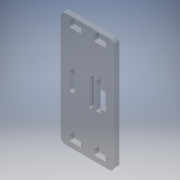
# Autodesk Inventor part: Front_wall
Saved by Autodesk Inventor 2016 (Build 200138000, 138)
## iProperties
Created: 2015-06-25
Part Number: Front_wall
Material: Generic
Document SubType Name: Modeling
Designer: Openlab
Density: 1 g/cm^3
Appearance: Polycarbonate - Clear
Author: Openlab
Autodesk Inventor part; units mm, degrees
ref_plane "YZ Plane" through (0, 0, 0) normal (1, 0, 0) x (0, 1, 0)
ref_plane "XZ Plane" through (0, 0, 0) normal (0, 1, 0) x (-1, 0, 0)
ref_plane "XY Plane" through (0, 0, 0) normal (0, 0, 1) x (1, 0, 0)
sketch "Sketch1" plane through (0, 0, 0) normal (0, 1, 0) x (-1, 0, 0)
  line L0 (15.75, -20.2435) -> (15.75, -42.6397) construction
  line L1 (13.2323, -33.5) -> (6.4845, -33.5) construction
  line L2 (31.5, -64) -> (31.5, -3)
  line L3 (0, -3) -> (0, -64)
  line L4 (28.5, 0) -> (3, 0)
  line L5 (3, -67) -> (28.5, -67)
  line L6 (14.8, -41) -> (13, -41)
  line L7 (13, -41) -> (13, -26)
  line L8 (13, -26) -> (14.8, -26)
  line L9 (14.8, -26) -> (14.8, -41)
  line L10 (26.5, -3) -> (19.5, -3)
  line L11 (19.5, -3) -> (19.5, -6)
  line L12 (19.5, -6) -> (26.5, -6)
  line L13 (26.5, -6) -> (26.5, -3)
  line L14 (12, -3) -> (5, -3)
  line L15 (5, -3) -> (5, -6)
  line L16 (5, -6) -> (12, -6)
  line L17 (12, -6) -> (12, -3)
  line L18 (26.5, -61) -> (19.5, -61)
  line L19 (19.5, -61) -> (19.5, -64)
  line L20 (19.5, -64) -> (26.5, -64)
  line L21 (26.5, -64) -> (26.5, -61)
  line L22 (12, -61) -> (5, -61)
  line L23 (5, -61) -> (5, -64)
  line L24 (5, -64) -> (12, -64)
  line L25 (12, -64) -> (12, -61)
  line L26 (8, -28.5) -> (5, -28.5)
  line L27 (5, -28.5) -> (5, -38.5)
  line L28 (5, -38.5) -> (8, -38.5)
  line L29 (8, -28.5) -> (8, -26)
  line L30 (8, -26) -> (11, -26)
  line L31 (11, -26) -> (11, -41)
  line L32 (11, -41) -> (8, -41)
  line L33 (8, -41) -> (8, -38.5)
  line L34 (26.5, -28.5) -> (23.5, -28.5)
  line L35 (23.5, -28.5) -> (23.5, -38.5)
  line L36 (23.5, -38.5) -> (26.5, -38.5)
  line L37 (26.5, -38.5) -> (26.5, -28.5)
  arc A0 (31.5, -3) -> (28.5, 0) centre (28.5, -3) ccw
  arc A1 (28.5, -67) -> (31.5, -64) centre (28.5, -64) ccw
  arc A2 (0, -64) -> (3, -67) centre (3, -64) ccw
  arc A3 (3, 0) -> (0, -3) centre (3, -3) ccw
  point P0 (0, 0)
  dimension "d22" = 15
  dimension "d24" = 1.8
  dimension "d27" = 7
  dimension "d28" = 3
  dimension "d29" = 5
  dimension "d30" = 3
  dimension "d31" = 7.5
  dimension "d32" = 13
  dimension "d33" = 10
  dimension "d34" = 15
  dimension "d35" = 6
  dimension "d36" = 31.5
  dimension "d37" = 67
  constraints: 76 end point, 15 parallel, 12 perpendicular, 10 point on line, 9 horizontal, 8 point on circle, 8 tangent, 7 equal length, 4 centre point, 3 equal radius, 2 collinear, 2 vertical, 7 other
  measures "d22" distance of L8.end L6.start
  measures "d24" distance of L7.end L8.end
  measures "d27" distance of L11.end L12.end
  measures "d28" distance of L14.end L15.end
  measures "d29" distance between parallel lines of L13 L2
  measures "d30" distance between parallel lines of L5 L24
  measures "d31" distance between parallel lines of L17 L11
  measures "d32" distance between parallel lines of L3 L7
  measures "d33" distance of L26.end L27.end
  measures "d34" distance of L30.end L31.end
  measures "d35" diameter of A0
  measures "d36" distance between parallel lines of L3 L2
  measures "d37" distance between parallel lines of L5 L4
extrude "Extrusion1" add sketch "Sketch1" along normal blind 3
body "Solid1"
